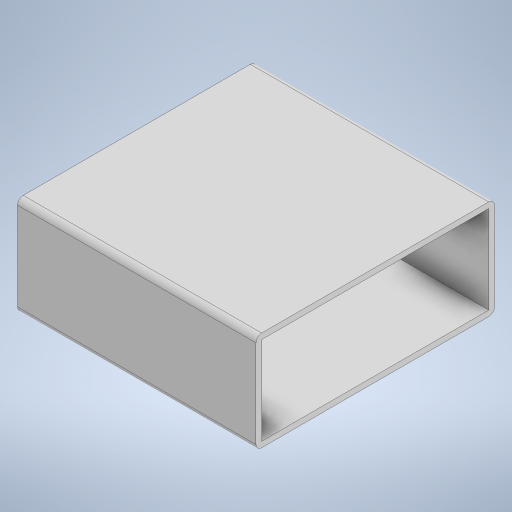
# Autodesk Inventor part: BatterieHolder
Saved by Autodesk Inventor 2023 (Build 270158000, 158)
## iProperties
Created: 2023-03-28
Part Number: BatterieHolder
Material: Générique
Document SubType Name: Modeling
Designer: eleves
Density: 1 g/cm^3
Appearance: Par défaut
Author: eleves
## iProperties of the stored document BatterieHolder_Impression 3D.ipt
Created: 2023-03-28
Part Number: BatterieHolder_Impression 3D
Material: Générique
Document SubType Name: Modeling
Designer: eleves
Density: 1 g/cm^3
Appearance: Par défaut
Author: eleves
Autodesk Inventor part; units mm, degrees
ref_plane "YZ Plane" through (0, 0, 0) normal (1, 0, 0) x (0, 1, 0)
ref_plane "XZ Plane" through (0, 0, 0) normal (0, 1, 0) x (-1, 0, 0)
ref_plane "XY Plane" through (0, 0, 0) normal (0, 0, 1) x (1, 0, 0)
sketch "Esquisse1" plane through (0, 0, 0) normal (0, 1, 0) x (-1, 0, 0)
  line L0 (-42, -42) -> (42, -42)
  line L1 (42, -42) -> (42, 42)
  line L2 (42, 42) -> (-42, 42)
  line L3 (-42, 42) -> (-42, -42)
  line L4 (-42, -42) -> (42, 42) construction
  line L5 (42, -42) -> (-42, 42) construction
  point P0 (0, 0)
  dimension "d0" = 84
  dimension "d1" = 84
  constraints: 12 end point, 2 midpoint, 2 parallel, 1 horizontal, 1 perpendicular
  measures "d0" distance between parallel lines of L0 L2
  measures "d1" distance of L1.end L2.end
extrude "Extrusion1" add sketch "Esquisse1" along normal blind 2
sketch "Esquisse2" plane through (0, 2, 0) normal (0, 1, 0) x (1, 0, 0)
  line L0 (40, 40) -> (-40, 40)
  line L1 (-40, 40) -> (-40, -40)
  line L2 (-40, -40) -> (40, -40)
  line L3 (40, 40) -> (-40, -40) construction
  line L4 (-40, 40) -> (40, -40) construction
  line L5 (40, -40) -> (42, -40)
  line L6 (42, -42) -> (42, 42) projected
  line L7 (40, 40) -> (42, 40)
  line L8 (-42, -42) -> (42, -42) projected
  line L9 (-42, 42) -> (-42, -42) projected
  line L10 (42, 42) -> (-42, 42) projected
  point P0 (0, 0)
  dimension "d4" = 2
  dimension "d5" = 2
  constraints: 14 end point, 2 horizontal, 2 midpoint, 2 perpendicular, 2 point on line, 1 parallel
  measures "d4" distance between parallel lines of L8 L2
  measures "d5" distance between parallel lines of L9 L1
extrude "Extrusion2" add sketch "Esquisse2" along normal blind 31 contours L0 L1 L2 L5 L6 L8 L9 L10 L7
sketch "Esquisse3" plane through (0, 33, 0) normal (0, 1, 0) x (1, 0, 0)
  line L0 (42, 40) -> (42, 42) projected
  line L1 (-42, -42) -> (42, -42)
  line L2 (42, -42) -> (42, 42)
  line L3 (42, 42) -> (-42, 42)
  line L4 (-42, 42) -> (-42, -42)
  point P0 (0, 0)
  constraints: 8 end point, 2 parallel, 1 horizontal, 1 perpendicular
extrude "Extrusion3" add sketch "Esquisse3" along normal blind 2
fillet "Congé1" radius 2 4 edges at (0, 35, 42) (0, 35, -42) (0, 0, 42) (0, 0, -42)
sketch "Esquisse5" plane through (-42, 0, -40) normal (-1, 0, 0) x (0, 0, 1)
  line L0 (40, 0) -> (40, 35.2291) construction
  circle A0 centre (40, 17.6146) radius 5
  dimension "d12" = 10
  constraints: 2 end point, 1 centre point, 1 midpoint, 1 vertical
  measures "d12" diameter of A0
extrude "Extrusion4" cut sketch "Esquisse5" against normal blind 31
